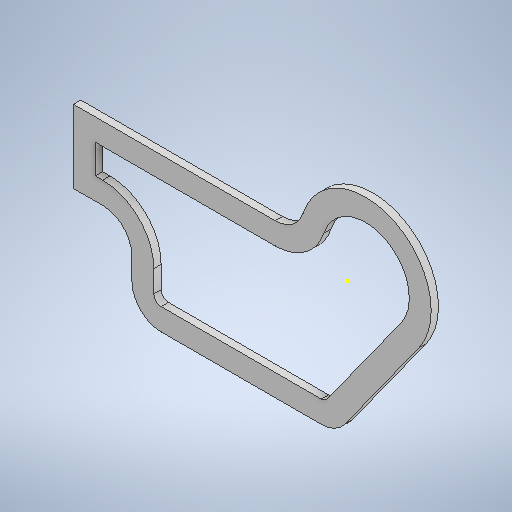
# Autodesk Inventor part: GASKET
Saved by Autodesk Inventor 2025.1 (Build 291241000, 241)
## iProperties
Created: 2024-11-14
Part Number: GASKET
Material: Generic
Document SubType Name: Modeling
Designer: bless
Density: 1 g/cm^3
Appearance: Default
Author: bless
Autodesk Inventor part; units mm, degrees
ref_plane "YZ Plane" through (0, 0, 0) normal (1, 0, 0) x (0, 1, 0)
ref_plane "XZ Plane" through (0, 0, 0) normal (0, 1, 0) x (-1, 0, 0)
ref_plane "XY Plane" through (0, 0, 0) normal (0, 0, 1) x (1, 0, 0)
sketch "Sketch1" plane through (0, 0, 0) normal (0, 0, 1) x (1, 0, 0)
  line L0 (-48.8466, 11.5644) -> (-187, 11.5644)
  line L1 (-187, 11.5644) -> (-187, -38.4356)
  line L2 (-187, -38.4356) -> (-167, -38.4356)
  line L3 (-147, -58.4356) -> (-147, -73.4356)
  line L4 (-127, -93.4356) -> (-17.2605, -93.4356)
  arc A0 (49.5519, -14.6836) -> (-29.8169, 25.4105) centre (13, 11.5644) ccw
  line L5 (49.5519, -14.6836) -> (-1.0152, -85.1014)
  arc A1 (-48.8466, 11.5644) -> (-29.8169, 25.4105) centre (-48.8466, 31.5644) ccw
  arc A2 (-147, -58.4356) -> (-167, -38.4356) centre (-167, -58.4356) ccw
  arc A3 (-147, -73.4356) -> (-127, -93.4356) centre (-127, -73.4356) ccw
  arc A4 (-17.2605, -93.4356) -> (-1.0152, -85.1014) centre (-17.2605, -73.4356) ccw
  point P0 (0, 0)
  point P1 (-32, 11.5644)
  point P2 (-147, -38.4356)
  point P3 (-147, -93.4356)
  point P4 (-7, -93.4356)
  dimension "d1" = 0
  dimension "d2" = 105
  dimension "d21" = 200
  dimension "d22" = 40
  dimension "d23" = 50
  dimension "d24" = 180
  dimension "d25" = 45
  dimension "d38" = 20
  dimension "d39" = 20
  constraints: 12 end point, 11 point on circle, 9 tangent, 7 point on line, 5 centre point, 4 perpendicular, 2 equal radius, 1 horizontal, 1 other
  measures "d1" distance from line of L0 A0.centre
  measures "d2" vertical distance of L0.end point (-147, -93.436)
  measures "d21" distance of L0.end A0.centre
  measures "d22" horizontal distance of point (-147, -93.436) L1.end
  measures "d23" vertical distance of point (-147, -38.436) L0.end
  measures "d24" horizontal distance of point (-7, -93.436) L1.end
  measures "d25" radius of A0
  measures "d38" radius of A1
  measures "d39" radius of A2
extrude "Extrusion1" add sketch "Sketch1" along normal blind 5
sketch "Sketch2" plane through (0, 0, 5) normal (0, 0, 1) x (1, 0, 0)
  arc A0 (-48.8466, 11.5644) -> (-29.8169, 25.4105) centre (-48.8466, 31.5644) ccw projected
  line L0 (-48.8466, 11.5644) -> (-187, 11.5644) projected
  line L1 (-187, 11.5644) -> (-187, -38.4356) projected
  line L2 (-187, -38.4356) -> (-167, -38.4356) projected
  arc A1 (-147, -58.4356) -> (-167, -38.4356) centre (-167, -58.4356) ccw projected
  line L3 (-147, -58.4356) -> (-147, -73.4356) projected
  arc A2 (-147, -73.4356) -> (-127, -93.4356) centre (-127, -73.4356) ccw projected
  line L4 (-127, -93.4356) -> (-17.2605, -93.4356) projected
  arc A3 (-17.2605, -93.4356) -> (-1.0152, -85.1014) centre (-17.2605, -73.4356) ccw projected
  line L5 (-1.0152, -85.1014) -> (49.5519, -14.6836) projected
  arc A4 (49.5519, -14.6836) -> (-29.8169, 25.4105) centre (13, 11.5644) ccw projected
  line L6 (-172, -3.4356) -> (-48.8466, -3.4356)
  arc A5 (-48.8466, -3.4356) -> (-15.5446, 20.7951) centre (-48.8466, 31.5644) ccw
  arc A6 (37.368, -5.9343) -> (-15.5446, 20.7951) centre (13, 11.5644) ccw
  line L7 (37.368, -5.9343) -> (-13.1992, -76.3521)
  arc A7 (-17.2605, -78.4356) -> (-13.1992, -76.3521) centre (-17.2605, -73.4356) ccw
  line L8 (-17.2605, -78.4356) -> (-127, -78.4356)
  arc A8 (-132, -73.4356) -> (-127, -78.4356) centre (-127, -73.4356) ccw
  line L9 (-132, -73.4356) -> (-132, -58.4356)
  arc A9 (-132, -58.4356) -> (-167, -23.4356) centre (-167, -58.4356) ccw
  line L10 (-167, -23.4356) -> (-172, -23.4356)
  line L11 (-172, -23.4356) -> (-172, -3.4356)
  point P0 (0, 0)
  dimension "d42" = 15
  constraints: 12 end point, 10 point on circle, 5 centre point, 10 other
  measures "d42" distance between parallel lines of L6 L0
extrude "Extrusion2" cut sketch "Sketch2" against normal through all contours L6 A5 A6 L7 A7 L8 A8 L9 A9 L10 L11
sketch "Sketch3" plane through (0, 0, 5) normal (0, 0, 1) x (1, 0, 0)
  point P0 (0, 0)
sketch "Sketch4" plane through (0, 0, 5) normal (0, 0, 1) x (1, 0, 0)
  point P0 (0, 0)
body "Solid1"
